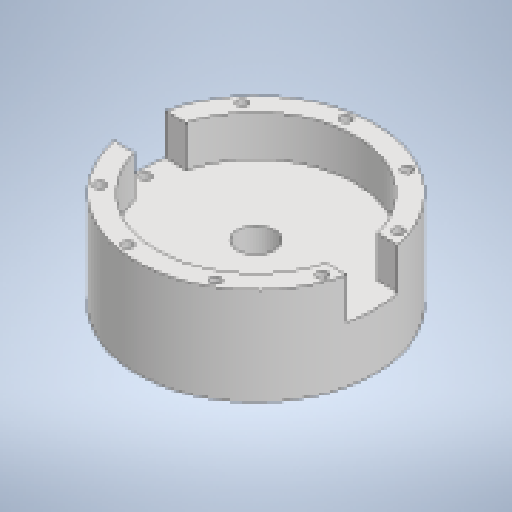
# Autodesk Inventor part: servofixpart_forR2
Saved by Autodesk Inventor 2024.3 (Build 283343010, 343A)
## iProperties
Created: 2025-05-25
Part Number: servofixpart_forR2
Material: 一般
Document SubType Name: Modeling
Designer: kshau
Density: 1 g/cm^3
Appearance: 既定
Mass: 104.118 g
Surface Area: 225.511 cm^2
Volume: 104.118 cm^3
Author: kshau
Autodesk Inventor part; units mm, degrees
ref_plane "YZ Plane" through (0, 0, 0) normal (1, 0, 0) x (0, 1, 0)
ref_plane "XZ Plane" through (0, 0, 0) normal (0, 1, 0) x (-1, 0, 0)
ref_plane "XY Plane" through (0, 0, 0) normal (0, 0, 1) x (1, 0, 0)
sketch "スケッチ1" plane through (0, 0, 0) normal (0, 1, 0) x (-1, 0, 0)
  circle A0 centre (0, 0) radius 39.25
  dimension "d0" = 78.5
  constraints: 1 centre point, 1 coincident
  measures "d0" diameter of A0
extrude "押し出し1" add sketch "スケッチ1" along normal blind 32
sketch "スケッチ2" plane through (0, 32, 0) normal (0, 1, 0) x (1, 0, 0)
  circle A0 centre (0, 0) radius 32.65
  dimension "d3" = 65.3
  constraints: 1 centre point, 1 coincident
  measures "d3" diameter of A0
extrude "押し出し2" cut sketch "スケッチ2" against normal blind 13.5
sketch "スケッチ3" plane through (0, 32, 0) normal (0, 1, 0) x (1, 0, 0)
  circle A0 centre (0, 0) radius 36.5
  point P0 (-36.5, 0)
  point P1 (-27.9606, -23.4617)
  point P2 (-6.3382, -35.9455)
  point P3 (18.25, -31.6099)
  point P4 (34.2988, -12.4837)
  point P5 (34.2988, 12.4837)
  point P6 (18.25, 31.6099)
  point P7 (-6.3382, 35.9455)
  point P8 (-27.9606, 23.4617)
  dimension "d6" = 73
  dimension "d9" = 360
  constraints: 1 coincident, 1 horizontal alignment, 12 other
hole "穴1" at (-36.5, 32, 0) at (-27.9606, 32, 23.4617) at (-6.3382, 32, 35.9455) at (18.25, 32, 31.6099) at (34.2988, 32, 12.4837) at (34.2988, 32, -12.4837) at (18.25, 32, -31.6099) at (-6.3382, 32, -35.9455) at (-27.9606, 32, -23.4617) direction (0, -1, 0) diameter 3.4 end through all
sketch "スケッチ4" plane through (0, 32, 0) normal (0, 1, 0) x (1, 0, 0)
  circle A0 centre (0, 0) radius 39.25 projected
  line L0 (38.3222, -8.4837) -> (-38.3222, -8.4837)
  line L1 (0, 0) -> (39.25, 0)
  circle A1 centre (34.2988, -12.4837) radius 1.7 projected
  line L2 (38.3222, 8.4837) -> (-38.3222, 8.4837)
  dimension "d18" = 4
  constraints: 6 end point, 3 point on circle, 2 horizontal, 2 symmetric about line, 1 parallel
  measures "d18" distance from line of A1.centre L0
extrude "押し出し3" cut sketch "スケッチ4" against normal blind 13.5 contours A0 L0 L2
sketch "スケッチ5" plane through (0, 18.5, 0) normal (0, 1, 0) x (1, 0, 0)
  circle A0 centre (-36.5, 0) radius 1.7 projected
  circle A1 centre (-36.5, 0) radius 3
  point P0 (0, 0)
  dimension "d21" = 6
  constraints: 1 centre point, 1 coincident
  measures "d21" diameter of A1
extrude "押し出し4" [suppressed]
sketch "スケッチ6" plane through (0, 0, 0) normal (0, -1, 0) x (1, 0, 0)
  circle A0 centre (0, 0) radius 15
  dimension "d24" = 30
  constraints: 1 centre point, 1 coincident
  measures "d24" diameter of A0
extrude "押し出し5" add sketch "スケッチ6" along normal blind 4
sketch "スケッチ7" plane through (0, -4, 0) normal (0, -1, 0) x (1, 0, 0)
  circle A0 centre (0, 0) radius 6
  dimension "d27" = 12
  constraints: 1 centre point, 1 coincident
  measures "d27" diameter of A0
extrude "押し出し6" cut sketch "スケッチ7" against normal blind 40
sketch "スケッチ8" plane through (0, -4, 0) normal (0, -1, 0) x (1, 0, 0)
  circle A0 centre (0, 0) radius 6 projected
  circle A1 centre (0, 0) radius 11
  dimension "d30" = 22
  constraints: 1 centre point, 1 coincident
  measures "d30" diameter of A1
extrude "押し出し7" cut sketch "スケッチ8" against normal blind 5
